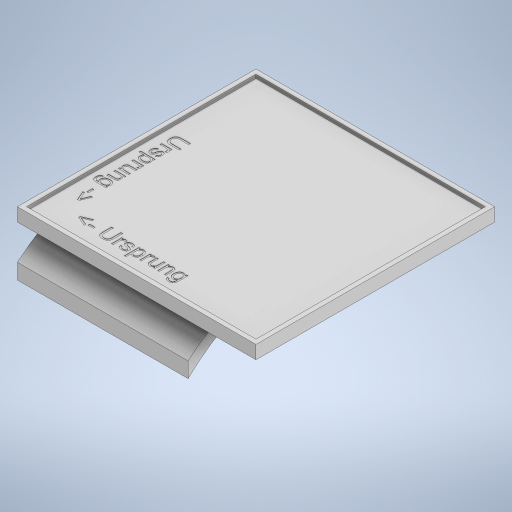
# Autodesk Inventor part: Arucomarkerhalterung
Saved by Autodesk Inventor 2024 (Build 280153000, 153)
## iProperties
Created: 2023-08-17
Part Number: Arucomarkerhalterung
Material: Generisch
Document SubType Name: Modeling
Designer: Jannik Eichmann
Density: 1 g/cm^3
Appearance: Vorgabe
Author: Jannik Eichmann
## iProperties of the stored document Arucomarkerhalterung_3D-Druck.ipt
Created: 2023-08-17
Part Number: Arucomarkerhalterung_3D-Druck
Material: Generisch
Document SubType Name: Modeling
Designer: Jannik Eichmann
Density: 1 g/cm^3
Appearance: Vorgabe
Author: Jannik Eichmann
Autodesk Inventor part; units mm, degrees
ref_plane "YZ Plane" through (0, 0, 0) normal (1, 0, 0) x (0, 1, 0)
ref_plane "XZ Plane" through (0, 0, 0) normal (0, 1, 0) x (-1, 0, 0)
ref_plane "XY Plane" through (0, 0, 0) normal (0, 0, 1) x (1, 0, 0)
sketch "Skizze1" plane through (0, 0, 0) normal (1, 0, 0) x (0, 1, 0)
  arc A0 (13.9194, -34.821) -> (13.9194, 34.821) centre (0, 0) ccw
  arc A1 (13.9194, -37.5) -> (13.9194, 37.5) centre (0, 0) ccw
  line L0 (13.9194, 37.5) -> (13.9194, -37.5)
  line L1 (36.1421, 10) -> (22.259, 10)
  line L2 (22.259, 10) -> (22.259, -10)
  line L3 (22.259, -10) -> (36.1421, -10)
  point P0 (27, -6)
  point P1 (27, 6)
  point P2 (40, 0)
  dimension "d0" = 75
  dimension "d1" = 80
  dimension "d4" = 13
  dimension "d5" = 13
  dimension "d6" = 6
  dimension "d7" = 6
  dimension "d8" = 20
  dimension "d22" = 10
  constraints: 8 end point, 7 point on circle, 2 centre point, 2 coincident, 2 point on line, 1 horizontal, 1 parallel, 1 perpendicular, 1 vertical
  measures "d0" diameter of A0
  measures "d1" diameter of A1
  measures "d4" horizontal distance of point (40, 0) point (27, 6)
  measures "d5" horizontal distance of point (40, 0) point (27, -6)
  measures "d6" vertical distance of point (40, 0) point (27, -6)
  measures "d7" vertical distance of point (27, 6) point (40, 0)
  measures "d8" distance of L2.end L1.end
  measures "d22" distance from line of point (40, 0) L1
extrude "Extrusion1" add sketch "Skizze1" along normal blind 37.2 contours A0 L0 A1
extrude "Extrusion2" add sketch "Skizze1" along normal blind 4 contours L3 L2 L1 A0
sketch "Skizze2" plane through (0, 0, 0) normal (-1, 0, 0) x (0, 0, 1)
  arc A0 (37.5, 13.9194) -> (-37.5, 13.9194) centre (0, 0) ccw projected
  point P0 (6, 27)
  point P1 (-6, 27)
  point P2 (0, 40)
  point P3 (0, 40)
  point P4 (0, 40)
  dimension "d24" = 13
  dimension "d25" = 13
  dimension "d26" = 6
  dimension "d27" = 12
  constraints: 3 point on circle
  measures "d24" vertical distance of point (-6, 27) point (0, 40)
  measures "d25" vertical distance of point (0, 40) point (6, 27)
  measures "d26" horizontal distance of point (0, 40) point (-6, 27)
  measures "d27" distance of point (6, 27) point (-6, 27)
hole "Bohrung1" at (0, 27, 6) at (0, 27, -6) direction (1, 0, 0) diameter 4.5 depth 54 tip angle 118
sketch "Skizze3" plane through (0, 0, 0) normal (-1, 0, 0) x (0, 0, 1)
  line L0 (-1, 40.0729) -> (-26, 40.0729)
  line L1 (-26, 40.0729) -> (-26, 37.9729)
  line L2 (-26, 37.9729) -> (-1, 37.9729)
  line L3 (-1, 37.9729) -> (-1, 40.0729)
  line L4 (-1, 40.0729) -> (26, 40.0729)
  line L5 (26, 40.0729) -> (26, 37.9729)
  line L6 (26, 37.9729) -> (-1, 37.9729)
  point P0 (0, 0)
  point P1 (26, 39.0229)
  dimension "d19" = 2.1
  dimension "d29" = 26
  dimension "d30" = 52
  constraints: 14 end point, 2 parallel, 1 horizontal, 1 midpoint, 1 perpendicular
  measures "d19" distance of L1.end L0.end
  measures "d29" horizontal distance of point (0, 0) point (26, 39.023)
  measures "d30" distance of L0.end L4.end
extrude "Extrusion3" add sketch "Skizze3" against normal blind 52
fillet "Rundung1" radius 4 2 edges at (2, 22.259, 10) (2, 22.259, -10)
fillet "Rundung2" radius 0.5 2 edges at (18.6, 37.9729, 12.5722) (18.6, 37.9729, -12.5722)
sketch "Skizze4" plane through (0, 40.0729, 26) normal (0, 1, 0) x (1, 0, 0)
  line L0 (0, 0) -> (52, 0) projected
  line L1 (52, 0) -> (52, 52) projected
  line L2 (0, 0) -> (52, 0)
  line L3 (52, 0) -> (52, 1)
  line L4 (51, 1) -> (1, 1)
  line L5 (0, 1) -> (0, 0)
  line L6 (0, 52) -> (52, 52) projected
  line L7 (0, 52) -> (1, 52)
  line L8 (1, 51) -> (1, 1)
  line L9 (1, 0) -> (0, 0)
  line L10 (0, 0) -> (0, 52)
  line L11 (52, 0) -> (51, 0)
  line L12 (51, 1) -> (51, 51)
  line L13 (51, 52) -> (52, 52)
  line L14 (52, 52) -> (52, 0)
  line L15 (0, 60.821) -> (0, 36) projected
  line L16 (52, 52) -> (0, 52)
  line L17 (0, 52) -> (0, 51)
  line L18 (1, 51) -> (51, 51)
  line L19 (52, 51) -> (52, 52)
  point P0 (0, 26)
  point P1 (0, 1)
  dimension "d33" = 1
  dimension "d34" = 1
  dimension "d35" = 1
  dimension "d36" = 1
  constraints: 32 end point, 8 parallel, 4 horizontal, 4 perpendicular, 4 point on line
  measures "d33" distance of L3.end L2.end
  measures "d34" distance of L9.start L9.end
  measures "d35" distance of L13.start L13.end
  measures "d36" distance of L17.end L16.end
extrude "Extrusion4" add sketch "Skizze4" along normal blind 0.8
sketch "Skizze5" plane through (1, 40.0729, 25) normal (0, 1, 0) x (1, 0, 0)
  line L0 (6.6345, 6.2294) -> (44.6715, 6.2294) construction
  line L1 (44.6715, 6.2294) -> (44.6715, 1.0918) construction
  line L2 (44.6715, 1.0918) -> (6.6345, 1.0918) construction
  line L3 (6.6345, 1.0918) -> (6.6345, 6.2294) construction
  line L4 (5.1531, 30.9392) -> (5.1531, 4.9173) construction
  line L5 (5.1531, 4.9173) -> (-0.6367, 4.9173) construction
  line L6 (-0.6367, 4.9173) -> (-0.6367, 30.9392) construction
  line L7 (-0.6367, 30.9392) -> (5.1531, 30.9392) construction
  line L8 (6.8761, 4.4463) -> (6.8761, 4.8111)
  line L9 (6.8761, 4.8111) -> (8.9734, 5.6979)
  line L10 (8.9734, 5.6979) -> (8.9734, 5.3089)
  line L11 (8.9734, 5.3089) -> (7.3111, 4.6275)
  line L12 (7.3111, 4.6275) -> (8.9734, 3.9389)
  line L13 (8.9734, 3.9389) -> (8.9734, 3.5499)
  line L14 (8.9734, 3.5499) -> (6.8761, 4.4463)
  line L15 (9.3575, 4.0114) -> (9.3575, 4.4028)
  line L16 (9.3575, 4.4028) -> (10.556, 4.4028)
  line L17 (10.556, 4.4028) -> (10.556, 4.0114)
  line L18 (10.556, 4.0114) -> (9.3575, 4.0114)
  line L19 (14.3445, 6.2294) -> (14.7649, 6.2294)
  line L20 (14.7649, 6.2294) -> (14.7649, 4.398)
  spline S0 degree 2 poles (14.7649, 4.398) (14.7649, 3.9196) (14.5499, 3.359) (13.9845, 3.0063) (13.5254, 3.0063) knots 0 0 0 1 2 3 3 3
  spline S1 degree 2 poles (13.5254, 3.0063) (13.0808, 3.0063) (12.513, 3.3131) (12.2714, 3.8954) (12.2714, 4.398) knots 0 0 0 1 2 3 3 3
  line L21 (12.2714, 4.398) -> (12.2714, 6.2294)
  line L22 (12.2714, 6.2294) -> (12.6918, 6.2294)
  line L23 (12.6918, 6.2294) -> (12.6918, 4.4004)
  spline S2 degree 2 poles (12.6918, 4.4004) (12.6918, 3.9896) (12.8441, 3.5982) (13.2186, 3.3856) (13.4892, 3.3856) knots 0 0 0 1 2 3 3 3
  spline S3 degree 2 poles (13.4892, 3.3856) (13.9507, 3.3856) (14.3445, 3.806) (14.3445, 4.4004) knots 0 0 0 1 2 2 2
  line L24 (14.3445, 4.4004) -> (14.3445, 6.2294)
  line L25 (15.41, 3.0594) -> (15.41, 5.3572)
  line L26 (15.41, 5.3572) -> (15.7604, 5.3572)
  line L27 (15.7604, 5.3572) -> (15.7604, 5.0093)
  spline S4 degree 2 poles (15.7604, 5.0093) (15.8932, 5.2533) (16.1204, 5.4079) (16.2581, 5.4079) knots 0 0 0 1 2 2 2
  spline S5 degree 2 poles (16.2581, 5.4079) (16.4538, 5.4079) (16.6568, 5.2847) knots 0 0 0 1 1 1
  line L28 (16.6568, 5.2847) -> (16.5214, 4.9223)
  spline S6 degree 2 poles (16.5214, 4.9223) (16.3789, 5.0069) (16.2363, 5.0069) knots 0 0 0 1 1 1
  spline S7 degree 2 poles (16.2363, 5.0069) (16.1083, 5.0069) (15.9077, 4.8522) (15.8643, 4.7169) knots 0 0 0 1 2 2 2
  spline S8 degree 2 poles (15.8643, 4.7169) (15.799, 4.5091) (15.799, 4.2627) knots 0 0 0 1 1 1
  line L29 (15.799, 4.2627) -> (15.799, 3.0594)
  line L30 (15.799, 3.0594) -> (15.41, 3.0594)
  line L31 (16.7317, 3.7456) -> (17.1158, 3.806)
  spline S9 degree 2 poles (17.1158, 3.806) (17.1472, 3.5741) (17.4444, 3.3276) (17.7126, 3.3276) knots 0 0 0 1 2 2 2
  spline S10 degree 2 poles (17.7126, 3.3276) (17.9808, 3.3276) (18.2418, 3.5475) (18.2418, 3.6949) knots 0 0 0 1 2 2 2
  spline S11 degree 2 poles (18.2418, 3.6949) (18.2418, 3.8253) (18.1258, 3.9027) knots 0 0 0 1 1 1
  spline S12 degree 2 poles (18.1258, 3.9027) (18.046, 3.9534) (17.7271, 4.0331) knots 0 0 0 1 1 1
  spline S13 degree 2 poles (17.7271, 4.0331) (17.2995, 4.1419) (16.9684, 4.2989) (16.7969, 4.5792) (16.7969, 4.7459) knots 0 0 0 1 2 3 3 3
  spline S14 degree 2 poles (16.7969, 4.7459) (16.7969, 4.9005) (16.937, 5.1615) (17.0578, 5.2485) knots 0 0 0 1 2 2 2
  spline S15 degree 2 poles (17.0578, 5.2485) (17.1496, 5.3161) (17.4638, 5.4079) (17.645, 5.4079) knots 0 0 0 1 2 2 2
  spline S16 degree 2 poles (17.645, 5.4079) (17.9156, 5.4079) (18.3239, 5.2509) (18.5196, 4.9851) (18.5559, 4.7628) knots 0 0 0 1 2 3 3 3
  line L32 (18.5559, 4.7628) -> (18.1741, 4.7121)
  spline S17 degree 2 poles (18.1741, 4.7121) (18.1475, 4.8909) (17.8987, 5.089) (17.6715, 5.089) knots 0 0 0 1 2 2 2
  spline S18 degree 2 poles (17.6715, 5.089) (17.4033, 5.089) (17.1738, 4.9102) (17.1738, 4.7918) knots 0 0 0 1 2 2 2
  spline S19 degree 2 poles (17.1738, 4.7918) (17.1738, 4.7169) (17.2221, 4.6565) knots 0 0 0 1 1 1
  spline S20 degree 2 poles (17.2221, 4.6565) (17.268, 4.5937) (17.3719, 4.5526) knots 0 0 0 1 1 1
  spline S21 degree 2 poles (17.3719, 4.5526) (17.4299, 4.5309) (17.715, 4.4511) knots 0 0 0 1 1 1
  spline S22 degree 2 poles (17.715, 4.4511) (18.1282, 4.3424) (18.4568, 4.2023) (18.6428, 3.9341) (18.6428, 3.7335) knots 0 0 0 1 2 3 3 3
  spline S23 degree 2 poles (18.6428, 3.7335) (18.6428, 3.5402) (18.4157, 3.1971) (17.9856, 3.0087) (17.715, 3.0087) knots 0 0 0 1 2 3 3 3
  spline S24 degree 2 poles (17.715, 3.0087) (17.268, 3.0087) (16.7969, 3.3808) (16.7317, 3.7456) knots 0 0 0 1 2 2 2
  line L33 (19.1043, 2.1799) -> (19.1043, 5.3572)
  line L34 (19.1043, 5.3572) -> (19.4595, 5.3572)
  line L35 (19.4595, 5.3572) -> (19.4595, 5.0576)
  spline S25 degree 2 poles (19.4595, 5.0576) (19.5851, 5.234) (19.8992, 5.4079) (20.1264, 5.4079) knots 0 0 0 1 2 2 2
  spline S26 degree 2 poles (20.1264, 5.4079) (20.4187, 5.4079) (20.8681, 5.1059) (21.0977, 4.555) (21.0977, 4.2264) knots 0 0 0 1 2 3 3 3
  spline S27 degree 2 poles (21.0977, 4.2264) (21.0977, 3.8737) (20.844, 3.3083) (20.3631, 3.0087) (20.0974, 3.0087) knots 0 0 0 1 2 3 3 3
  spline S28 degree 2 poles (20.0974, 3.0087) (19.9017, 3.0087) (19.5924, 3.173) (19.4933, 3.2986) knots 0 0 0 1 2 2 2
  line L36 (19.4933, 3.2986) -> (19.4933, 2.1799)
  line L37 (19.4933, 2.1799) -> (19.1043, 2.1799)
  spline S29 degree 2 poles (19.4571, 4.195) (19.4571, 3.7504) (19.8147, 3.3276) (20.0684, 3.3276) knots 0 0 0 1 2 2 2
  spline S30 degree 2 poles (20.0684, 3.3276) (20.3269, 3.3276) (20.6966, 3.7674) (20.6966, 4.2264) knots 0 0 0 1 2 2 2
  spline S31 degree 2 poles (20.6966, 4.2264) (20.6966, 4.6662) (20.3366, 5.1035) (20.0877, 5.1035) knots 0 0 0 1 2 2 2
  spline S32 degree 2 poles (20.0877, 5.1035) (19.8388, 5.1035) (19.4571, 4.6396) (19.4571, 4.195) knots 0 0 0 1 2 2 2
  line L38 (21.5616, 3.0594) -> (21.5616, 5.3572)
  line L39 (21.5616, 5.3572) -> (21.9119, 5.3572)
  line L40 (21.9119, 5.3572) -> (21.9119, 5.0093)
  spline S33 degree 2 poles (21.9119, 5.0093) (22.0448, 5.2533) (22.2719, 5.4079) (22.4096, 5.4079) knots 0 0 0 1 2 2 2
  spline S34 degree 2 poles (22.4096, 5.4079) (22.6053, 5.4079) (22.8083, 5.2847) knots 0 0 0 1 1 1
  line L41 (22.8083, 5.2847) -> (22.673, 4.9223)
  spline S35 degree 2 poles (22.673, 4.9223) (22.5304, 5.0069) (22.3879, 5.0069) knots 0 0 0 1 1 1
  spline S36 degree 2 poles (22.3879, 5.0069) (22.2598, 5.0069) (22.0593, 4.8522) (22.0158, 4.7169) knots 0 0 0 1 2 2 2
  spline S37 degree 2 poles (22.0158, 4.7169) (21.9506, 4.5091) (21.9506, 4.2627) knots 0 0 0 1 1 1
  line L42 (21.9506, 4.2627) -> (21.9506, 3.0594)
  line L43 (21.9506, 3.0594) -> (21.5616, 3.0594)
  line L44 (24.5431, 3.0594) -> (24.5431, 3.3977)
  spline S38 degree 2 poles (24.5431, 3.3977) (24.2749, 3.0087) (23.8158, 3.0087) knots 0 0 0 1 1 1
  spline S39 degree 2 poles (23.8158, 3.0087) (23.6129, 3.0087) (23.2601, 3.1633) (23.0886, 3.4001) (23.0547, 3.5717) knots 0 0 0 1 2 3 3 3
  spline S40 degree 2 poles (23.0547, 3.5717) (23.0306, 3.6852) (23.0306, 3.9341) knots 0 0 0 1 1 1
  line L45 (23.0306, 3.9341) -> (23.0306, 5.3572)
  line L46 (23.0306, 5.3572) -> (23.4196, 5.3572)
  line L47 (23.4196, 5.3572) -> (23.4196, 4.0839)
  spline S41 degree 2 poles (23.4196, 4.0839) (23.4196, 3.7794) (23.4437, 3.6731) knots 0 0 0 1 1 1
  spline S42 degree 2 poles (23.4437, 3.6731) (23.48, 3.5185) (23.7168, 3.3445) (23.8931, 3.3445) knots 0 0 0 1 2 2 2
  spline S43 degree 2 poles (23.8931, 3.3445) (24.0671, 3.3445) (24.374, 3.5233) (24.502, 3.8326) (24.502, 4.1274) knots 0 0 0 1 2 3 3 3
  line L48 (24.502, 4.1274) -> (24.502, 5.3572)
  line L49 (24.502, 5.3572) -> (24.891, 5.3572)
  line L50 (24.891, 5.3572) -> (24.891, 3.0594)
  line L51 (24.891, 3.0594) -> (24.5431, 3.0594)
  line L52 (25.5023, 3.0594) -> (25.5023, 5.3572)
  line L53 (25.5023, 5.3572) -> (25.8527, 5.3572)
  line L54 (25.8527, 5.3572) -> (25.8527, 5.031)
  spline S44 degree 2 poles (25.8527, 5.031) (26.1063, 5.4079) (26.5823, 5.4079) knots 0 0 0 1 1 1
  spline S45 degree 2 poles (26.5823, 5.4079) (26.7901, 5.4079) (27.138, 5.2581) (27.312, 5.0165) (27.3458, 4.8498) knots 0 0 0 1 2 3 3 3
  spline S46 degree 2 poles (27.3458, 4.8498) (27.3676, 4.7411) (27.3676, 4.4705) knots 0 0 0 1 1 1
  line L55 (27.3676, 4.4705) -> (27.3676, 3.0594)
  line L56 (27.3676, 3.0594) -> (26.9786, 3.0594)
  line L57 (26.9786, 3.0594) -> (26.9786, 4.456)
  spline S47 degree 2 poles (26.9786, 4.456) (26.9786, 4.6928) (26.8868, 4.9295) (26.6572, 5.0697) (26.5002, 5.0697) knots 0 0 0 1 2 3 3 3
  spline S48 degree 2 poles (26.5002, 5.0697) (26.2513, 5.0697) (25.8913, 4.7532) (25.8913, 4.3134) knots 0 0 0 1 2 2 2
  line L58 (25.8913, 4.3134) -> (25.8913, 3.0594)
  line L59 (25.8913, 3.0594) -> (25.5023, 3.0594)
  line L60 (27.8919, 2.871) -> (28.2712, 2.8154)
  spline S49 degree 2 poles (28.2712, 2.8154) (28.2954, 2.639) (28.4041, 2.5593) knots 0 0 0 1 1 1
  spline S50 degree 2 poles (28.4041, 2.5593) (28.5491, 2.4506) (28.8004, 2.4506) knots 0 0 0 1 1 1
  spline S51 degree 2 poles (28.8004, 2.4506) (29.0686, 2.4506) (29.3633, 2.6656) (29.4165, 2.8613) knots 0 0 0 1 2 2 2
  spline S52 degree 2 poles (29.4165, 2.8613) (29.4455, 2.9797) (29.4431, 3.359) knots 0 0 0 1 1 1
  spline S53 degree 2 poles (29.4431, 3.359) (29.1894, 3.0594) (28.8076, 3.0594) knots 0 0 0 1 1 1
  spline S54 degree 2 poles (28.8076, 3.0594) (28.334, 3.0594) (27.8146, 3.7432) (27.8146, 4.2216) knots 0 0 0 1 2 2 2
  spline S55 degree 2 poles (27.8146, 4.2216) (27.8146, 4.5502) (28.0538, 5.1059) (28.5056, 5.4079) (28.81, 5.4079) knots 0 0 0 1 2 3 3 3
  spline S56 degree 2 poles (28.81, 5.4079) (29.2159, 5.4079) (29.4793, 5.0793) knots 0 0 0 1 1 1
  line L61 (29.4793, 5.0793) -> (29.4793, 5.3572)
  line L62 (29.4793, 5.3572) -> (29.8393, 5.3572)
  line L63 (29.8393, 5.3572) -> (29.8393, 3.3735)
  spline S57 degree 2 poles (29.8393, 3.3735) (29.8393, 2.8371) (29.6219, 2.3877) (29.1483, 2.1292) (28.8004, 2.1292) knots 0 0 0 1 2 3 3 3
  spline S58 degree 2 poles (28.8004, 2.1292) (28.3896, 2.1292) (27.8846, 2.4989) (27.8919, 2.871) knots 0 0 0 1 2 2 2
  spline S59 degree 2 poles (28.2157, 4.2482) (28.2157, 3.7964) (28.5757, 3.3808) (28.8439, 3.3808) knots 0 0 0 1 2 2 2
  spline S60 degree 2 poles (28.8439, 3.3808) (29.1121, 3.3808) (29.4745, 3.7939) (29.4745, 4.2361) knots 0 0 0 1 2 2 2
  spline S61 degree 2 poles (29.4745, 4.2361) (29.4745, 4.6589) (29.1024, 5.0866) (28.839, 5.0866) knots 0 0 0 1 2 2 2
  spline S62 degree 2 poles (28.839, 5.0866) (28.5781, 5.0866) (28.2157, 4.6638) (28.2157, 4.2482) knots 0 0 0 1 2 2 2
  line L64 (5.1531, 28.5182) -> (5.1531, 28.0978)
  line L65 (5.1531, 28.0978) -> (3.3216, 28.0978)
  spline S63 degree 2 poles (3.3216, 28.0978) (2.8432, 28.0978) (2.2827, 28.3128) (1.9299, 28.8782) (1.9299, 29.3373) knots 0 0 0 1 2 3 3 3
  spline S64 degree 2 poles (1.9299, 29.3373) (1.9299, 29.7818) (2.2368, 30.3496) (2.8191, 30.5912) (3.3216, 30.5912) knots 0 0 0 1 2 3 3 3
  line L66 (3.3216, 30.5912) -> (5.1531, 30.5912)
  line L67 (5.1531, 30.5912) -> (5.1531, 30.1708)
  line L68 (5.1531, 30.1708) -> (3.324, 30.1708)
  spline S65 degree 2 poles (3.324, 30.1708) (2.9133, 30.1708) (2.5219, 30.0186) (2.3093, 29.6441) (2.3093, 29.3735) knots 0 0 0 1 2 3 3 3
  spline S66 degree 2 poles (2.3093, 29.3735) (2.3093, 28.912) (2.7297, 28.5182) (3.324, 28.5182) knots 0 0 0 1 2 2 2
  line L69 (3.324, 28.5182) -> (5.1531, 28.5182)
  line L70 (1.9831, 27.4527) -> (4.2808, 27.4527)
  line L71 (4.2808, 27.4527) -> (4.2808, 27.1023)
  line L72 (4.2808, 27.1023) -> (3.9329, 27.1023)
  spline S67 degree 2 poles (3.9329, 27.1023) (4.1769, 26.9694) (4.3316, 26.7423) (4.3316, 26.6046) knots 0 0 0 1 2 2 2
  spline S68 degree 2 poles (4.3316, 26.6046) (4.3316, 26.4089) (4.2084, 26.2059) knots 0 0 0 1 1 1
  line L73 (4.2084, 26.2059) -> (3.8459, 26.3412)
  spline S69 degree 2 poles (3.8459, 26.3412) (3.9305, 26.4838) (3.9305, 26.6263) knots 0 0 0 1 1 1
  spline S70 degree 2 poles (3.9305, 26.6263) (3.9305, 26.7544) (3.7759, 26.9549) (3.6406, 26.9984) knots 0 0 0 1 2 2 2
  spline S71 degree 2 poles (3.6406, 26.9984) (3.4328, 27.0637) (3.1863, 27.0637) knots 0 0 0 1 1 1
  line L74 (3.1863, 27.0637) -> (1.9831, 27.0637)
  line L75 (1.9831, 27.0637) -> (1.9831, 27.4527)
  line L76 (2.6693, 26.131) -> (2.7297, 25.7469)
  spline S72 degree 2 poles (2.7297, 25.7469) (2.4977, 25.7154) (2.2513, 25.4183) (2.2513, 25.1501) knots 0 0 0 1 2 2 2
  spline S73 degree 2 poles (2.2513, 25.1501) (2.2513, 24.8819) (2.4711, 24.6209) (2.6185, 24.6209) knots 0 0 0 1 2 2 2
  spline S74 degree 2 poles (2.6185, 24.6209) (2.749, 24.6209) (2.8263, 24.7369) knots 0 0 0 1 1 1
  spline S75 degree 2 poles (2.8263, 24.7369) (2.8771, 24.8166) (2.9568, 25.1356) knots 0 0 0 1 1 1
  spline S76 degree 2 poles (2.9568, 25.1356) (3.0655, 25.5632) (3.2226, 25.8942) (3.5028, 26.0658) (3.6696, 26.0658) knots 0 0 0 1 2 3 3 3
  spline S77 degree 2 poles (3.6696, 26.0658) (3.8242, 26.0658) (4.0851, 25.9256) (4.1721, 25.8048) knots 0 0 0 1 2 2 2
  spline S78 degree 2 poles (4.1721, 25.8048) (4.2398, 25.713) (4.3316, 25.3989) (4.3316, 25.2177) knots 0 0 0 1 2 2 2
  spline S79 degree 2 poles (4.3316, 25.2177) (4.3316, 24.9471) (4.1745, 24.5388) (3.9087, 24.3431) (3.6865, 24.3068) knots 0 0 0 1 2 3 3 3
  line L77 (3.6865, 24.3068) -> (3.6357, 24.6886)
  spline S80 degree 2 poles (3.6357, 24.6886) (3.8145, 24.7152) (4.0126, 24.964) (4.0126, 25.1911) knots 0 0 0 1 2 2 2
  spline S81 degree 2 poles (4.0126, 25.1911) (4.0126, 25.4593) (3.8338, 25.6889) (3.7155, 25.6889) knots 0 0 0 1 2 2 2
  spline S82 degree 2 poles (3.7155, 25.6889) (3.6406, 25.6889) (3.5802, 25.6405) knots 0 0 0 1 1 1
  spline S83 degree 2 poles (3.5802, 25.6405) (3.5173, 25.5946) (3.4763, 25.4907) knots 0 0 0 1 1 1
  spline S84 degree 2 poles (3.4763, 25.4907) (3.4545, 25.4328) (3.3748, 25.1476) knots 0 0 0 1 1 1
  spline S85 degree 2 poles (3.3748, 25.1476) (3.2661, 24.7345) (3.1259, 24.4059) (2.8577, 24.2198) (2.6572, 24.2198) knots 0 0 0 1 2 3 3 3
  spline S86 degree 2 poles (2.6572, 24.2198) (2.4639, 24.2198) (2.1208, 24.447) (1.9323, 24.877) (1.9323, 25.1476) knots 0 0 0 1 2 3 3 3
  spline S87 degree 2 poles (1.9323, 25.1476) (1.9323, 25.5946) (2.3044, 26.0658) (2.6693, 26.131) knots 0 0 0 1 2 2 2
  line L78 (1.1036, 23.7584) -> (4.2808, 23.7584)
  line L79 (4.2808, 23.7584) -> (4.2808, 23.4032)
  line L80 (4.2808, 23.4032) -> (3.9812, 23.4032)
  spline S88 degree 2 poles (3.9812, 23.4032) (4.1576, 23.2775) (4.3316, 22.9634) (4.3316, 22.7363) knots 0 0 0 1 2 2 2
  spline S89 degree 2 poles (4.3316, 22.7363) (4.3316, 22.444) (4.0296, 21.9946) (3.4787, 21.765) (3.1501, 21.765) knots 0 0 0 1 2 3 3 3
  spline S90 degree 2 poles (3.1501, 21.765) (2.7973, 21.765) (2.2319, 22.0187) (1.9323, 22.4995) (1.9323, 22.7653) knots 0 0 0 1 2 3 3 3
  spline S91 degree 2 poles (1.9323, 22.7653) (1.9323, 22.961) (2.0966, 23.2703) (2.2223, 23.3694) knots 0 0 0 1 2 2 2
  line L81 (2.2223, 23.3694) -> (1.1036, 23.3694)
  line L82 (1.1036, 23.3694) -> (1.1036, 23.7584)
  spline S92 degree 2 poles (3.1187, 23.4056) (2.6741, 23.4056) (2.2513, 23.048) (2.2513, 22.7943) knots 0 0 0 1 2 2 2
  spline S93 degree 2 poles (2.2513, 22.7943) (2.2513, 22.5358) (2.691, 22.1661) (3.1501, 22.1661) knots 0 0 0 1 2 2 2
  spline S94 degree 2 poles (3.1501, 22.1661) (3.5898, 22.1661) (4.0271, 22.5261) (4.0271, 22.775) knots 0 0 0 1 2 2 2
  spline S95 degree 2 poles (4.0271, 22.775) (4.0271, 23.0238) (3.5632, 23.4056) (3.1187, 23.4056) knots 0 0 0 1 2 2 2
  line L83 (1.9831, 21.3011) -> (4.2808, 21.3011)
  line L84 (4.2808, 21.3011) -> (4.2808, 20.9508)
  line L85 (4.2808, 20.9508) -> (3.9329, 20.9508)
  spline S96 degree 2 poles (3.9329, 20.9508) (4.1769, 20.8179) (4.3316, 20.5908) (4.3316, 20.453) knots 0 0 0 1 2 2 2
  spline S97 degree 2 poles (4.3316, 20.453) (4.3316, 20.2573) (4.2084, 20.0544) knots 0 0 0 1 1 1
  line L86 (4.2084, 20.0544) -> (3.8459, 20.1897)
  spline S98 degree 2 poles (3.8459, 20.1897) (3.9305, 20.3322) (3.9305, 20.4748) knots 0 0 0 1 1 1
  spline S99 degree 2 poles (3.9305, 20.4748) (3.9305, 20.6029) (3.7759, 20.8034) (3.6406, 20.8469) knots 0 0 0 1 2 2 2
  spline S100 degree 2 poles (3.6406, 20.8469) (3.4328, 20.9121) (3.1863, 20.9121) knots 0 0 0 1 1 1
  line L87 (3.1863, 20.9121) -> (1.9831, 20.9121)
  line L88 (1.9831, 20.9121) -> (1.9831, 21.3011)
  line L89 (1.9831, 18.3196) -> (2.3213, 18.3196)
  spline S101 degree 2 poles (2.3213, 18.3196) (1.9323, 18.5878) (1.9323, 19.0468) knots 0 0 0 1 1 1
  spline S102 degree 2 poles (1.9323, 19.0468) (1.9323, 19.2498) (2.087, 19.6026) (2.3237, 19.7741) (2.4953, 19.8079) knots 0 0 0 1 2 3 3 3
  spline S103 degree 2 poles (2.4953, 19.8079) (2.6089, 19.8321) (2.8577, 19.8321) knots 0 0 0 1 1 1
  line L90 (2.8577, 19.8321) -> (4.2808, 19.8321)
  line L91 (4.2808, 19.8321) -> (4.2808, 19.4431)
  line L92 (4.2808, 19.4431) -> (3.0075, 19.4431)
  spline S104 degree 2 poles (3.0075, 19.4431) (2.7031, 19.4431) (2.5968, 19.4189) knots 0 0 0 1 1 1
  spline S105 degree 2 poles (2.5968, 19.4189) (2.4421, 19.3827) (2.2682, 19.1459) (2.2682, 18.9695) knots 0 0 0 1 2 2 2
  spline S106 degree 2 poles (2.2682, 18.9695) (2.2682, 18.7956) (2.447, 18.4887) (2.7562, 18.3607) (3.051, 18.3607) knots 0 0 0 1 2 3 3 3
  line L93 (3.051, 18.3607) -> (4.2808, 18.3607)
  line L94 (4.2808, 18.3607) -> (4.2808, 17.9717)
  line L95 (4.2808, 17.9717) -> (1.9831, 17.9717)
  line L96 (1.9831, 17.9717) -> (1.9831, 18.3196)
  line L97 (1.9831, 17.3604) -> (4.2808, 17.3604)
  line L98 (4.2808, 17.3604) -> (4.2808, 17.01)
  line L99 (4.2808, 17.01) -> (3.9547, 17.01)
  spline S107 degree 2 poles (3.9547, 17.01) (4.3316, 16.7563) (4.3316, 16.2803) knots 0 0 0 1 1 1
  spline S108 degree 2 poles (4.3316, 16.2803) (4.3316, 16.0726) (4.1818, 15.7246) (3.9402, 15.5507) (3.7734, 15.5168) knots 0 0 0 1 2 3 3 3
  spline S109 degree 2 poles (3.7734, 15.5168) (3.6647, 15.4951) (3.3941, 15.4951) knots 0 0 0 1 1 1
  line L100 (3.3941, 15.4951) -> (1.9831, 15.4951)
  line L101 (1.9831, 15.4951) -> (1.9831, 15.8841)
  line L102 (1.9831, 15.8841) -> (3.3796, 15.8841)
  spline S110 degree 2 poles (3.3796, 15.8841) (3.6164, 15.8841) (3.8532, 15.9759) (3.9933, 16.2054) (3.9933, 16.3625) knots 0 0 0 1 2 3 3 3
  spline S111 degree 2 poles (3.9933, 16.3625) (3.9933, 16.6114) (3.6768, 16.9714) (3.2371, 16.9714) knots 0 0 0 1 2 2 2
  line L103 (3.2371, 16.9714) -> (1.9831, 16.9714)
  line L104 (1.9831, 16.9714) -> (1.9831, 17.3604)
  line L105 (1.7946, 14.9708) -> (1.739, 14.5914)
  spline S112 degree 2 poles (1.739, 14.5914) (1.5627, 14.5673) (1.4829, 14.4586) knots 0 0 0 1 1 1
  spline S113 degree 2 poles (1.4829, 14.4586) (1.3742, 14.3136) (1.3742, 14.0623) knots 0 0 0 1 1 1
  spline S114 degree 2 poles (1.3742, 14.0623) (1.3742, 13.7941) (1.5892, 13.4993) (1.7849, 13.4462) knots 0 0 0 1 2 2 2
  spline S115 degree 2 poles (1.7849, 13.4462) (1.9033, 13.4172) (2.2827, 13.4196) knots 0 0 0 1 1 1
  spline S116 degree 2 poles (2.2827, 13.4196) (1.9831, 13.6733) (1.9831, 14.0551) knots 0 0 0 1 1 1
  spline S117 degree 2 poles (1.9831, 14.0551) (1.9831, 14.5286) (2.6668, 15.0481) (3.1452, 15.0481) knots 0 0 0 1 2 2 2
  spline S118 degree 2 poles (3.1452, 15.0481) (3.4738, 15.0481) (4.0296, 14.8089) (4.3316, 14.3571) (4.3316, 14.0526) knots 0 0 0 1 2 3 3 3
  spline S119 degree 2 poles (4.3316, 14.0526) (4.3316, 13.6467) (4.003, 13.3834) knots 0 0 0 1 1 1
  line L106 (4.003, 13.3834) -> (4.2808, 13.3834)
  line L107 (4.2808, 13.3834) -> (4.2808, 13.0234)
  line L108 (4.2808, 13.0234) -> (2.2972, 13.0234)
  spline S120 degree 2 poles (2.2972, 13.0234) (1.7608, 13.0234) (1.3114, 13.2408) (1.0529, 13.7144) (1.0529, 14.0623) knots 0 0 0 1 2 3 3 3
  spline S121 degree 2 poles (1.0529, 14.0623) (1.0529, 14.4731) (1.4225, 14.978) (1.7946, 14.9708) knots 0 0 0 1 2 2 2
  spline S122 degree 2 poles (3.1718, 14.647) (2.72, 14.647) (2.3044, 14.287) (2.3044, 14.0188) knots 0 0 0 1 2 2 2
  spline S123 degree 2 poles (2.3044, 14.0188) (2.3044, 13.7506) (2.7176, 13.3882) (3.1597, 13.3882) knots 0 0 0 1 2 2 2
  spline S124 degree 2 poles (3.1597, 13.3882) (3.5826, 13.3882) (4.0102, 13.7603) (4.0102, 14.0237) knots 0 0 0 1 2 2 2
  spline S125 degree 2 poles (4.0102, 14.0237) (4.0102, 14.2846) (3.5874, 14.647) (3.1718, 14.647) knots 0 0 0 1 2 2 2
  line L109 (2.935, 11.361) -> (3.3265, 11.361)
  line L110 (3.3265, 11.361) -> (3.3265, 10.1626)
  line L111 (3.3265, 10.1626) -> (2.935, 10.1626)
  line L112 (2.935, 10.1626) -> (2.935, 11.361)
  line L113 (3.3699, 7.6861) -> (2.4736, 9.7833)
  line L114 (2.4736, 9.7833) -> (2.8626, 9.7833)
  line L115 (2.8626, 9.7833) -> (3.5512, 8.1234)
  line L116 (3.5512, 8.1234) -> (4.2325, 9.7833)
  line L117 (4.2325, 9.7833) -> (4.6215, 9.7833)
  line L118 (4.6215, 9.7833) -> (3.7348, 7.6861)
  line L119 (3.7348, 7.6861) -> (3.3699, 7.6861)
  point P0 (-1, 25)
  constraints: 4 other
emboss "Prägen1" sketch "Skizze5" operation cut depth 0.1 direction (0, -1, 0)
sketch "Skizze6" plane through (37.2, 0, 0) normal (1, 0, 0) x (0, 0, -1)
  line L0 (-15.3634, 37.9729) -> (-26, 37.9729) projected
  line L1 (-26, 37.9729) -> (-26, 21.1668)
  line L2 (-26, 21.1668) -> (-35.0972, 8.3823)
  line L3 (-35.0972, 8.3823) -> (-46.8873, 16.7719)
  line L4 (-46.8873, 16.7719) -> (-37.7901, 29.5564)
  line L5 (-37.7901, 29.5564) -> (-26, 33.6462)
  line L6 (26, 37.9729) -> (26, 40.8729) projected
  line L7 (26, 37.9729) -> (26, 23.1641)
  line L8 (26, 23.1641) -> (34.3735, 7.0556)
  line L9 (34.3735, 7.0556) -> (45.7107, 9.4678)
  line L10 (45.7107, 9.4678) -> (41.681, 21.0848)
  line L11 (41.681, 21.0848) -> (26, 33.6462)
  point P0 (0, 0)
  constraints: 20 end point, 3 perpendicular, 2 point on line, 2 vertical
extrude "Extrusion5" cut sketch "Skizze6" against normal blind 50
